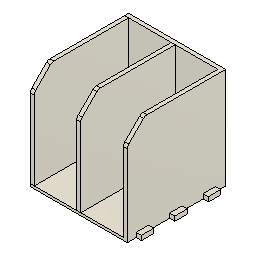
Centerpiece Divider Rack (Autodesk Fusion 360 design; units mm, degrees)
Autodesk Fusion 360 part; units mm, degrees
sketch "Base" plane through (0, 0, 0) normal (0, 1, 0) x (1, 0, 0) in component "DDD Wall Control Center Piece Parametric Template"
  line L0 (36.995, -37.5) -> (-36.995, -37.5)
  line L1 (-36.995, -37.5) -> (-36.995, 37.5)
  line L2 (-36.995, 37.5) -> (36.995, 37.5)
  line L3 (36.995, 37.5) -> (36.995, -37.5)
  line L4 (36.995, -37.5) -> (-36.995, 37.5) construction
  line L5 (-36.995, -37.5) -> (36.995, 37.5) construction
  dimension "d1" = 73.99
  dimension "d2" = 75
  constraint horizontal L0
  constraint perpendicular L0 L1
  constraint parallel L0 L2
  constraint parallel L1 L3
  constraint coincident L4 origin
  constraint coincident L5 origin
  constraint vertical L1
  measures "d1" distance of L1.end L2.end
  measures "d2" distance of L0.end L1.end
extrude "Extrude1" add sketch "Base" along normal blind 2 makes body 1 in component "DDD Wall Control Center Piece Parametric Template"
sketch "Mouting Tab" plane through (0, 0, 0) normal (1, 0, 0) x (0, 0, 1) in component "DDD Wall Control Center Piece Parametric Template"
  line L0 (-20.25, -3.5) -> (-29.75, -3.5)
  line L1 (-29.75, -3.5) -> (-29.75, 0)
  line L2 (-29.75, 0) -> (-20.25, 0)
  line L3 (-20.25, 0) -> (-20.25, -3.5)
  line L4 (-20.25, -3.5) -> (-29.75, 0) construction
  line L5 (-29.75, -3.5) -> (-20.25, 0) construction
  line L6 (1.75, 0) -> (22.5, 0)
  point P0 (-25, -1.75)
  dimension "d34" = 9.5
  dimension "d35" = 3.5
  dimension "d147" = 20.25
  constraint horizontal L0
  constraint perpendicular L0 L1
  constraint parallel L0 L2
  constraint parallel L1 L3
  constraint coincident L4 P0
  constraint coincident L5 P0
  constraint collinear L2 L6
  measures "d34" distance of L1.end L2.end
  measures "d35" distance of L0.end L1.end
  measures "d147" horizontal distance of L2.end origin
extrude "Extrude3" add sketch "Mouting Tab" along normal blind 4 from surface at 36.995 bodies 1 in component "DDD Wall Control Center Piece Parametric Template"
extrude "Extrude6" add sketch "Mouting Tab" against normal blind 4 from surface at -36.995 bodies 1 in component "DDD Wall Control Center Piece Parametric Template"
pattern_linear "R-Pattern2" count 1 spacing 177.59 along (0, -1, 0) count 3 spacing 25.5 along (0, 0, 1) of "Extrude3", "Extrude6" in component "DDD Wall Control Center Piece Parametric Template"
sketch "Side and Back Walls" plane through (0, 2, 0) normal (0, 1, 0) x (-1, 0, 0) in component "DDD Wall Control Center Piece Parametric Template"
  line L0 (-36.995, -37.5) -> (36.995, -37.5)
  line L1 (36.995, -37.5) -> (36.995, 37.5)
  line L2 (36.995, 37.5) -> (-36.995, 37.5)
  line L3 (-36.995, 37.5) -> (-36.995, 30.75)
  line L4 (36.995, -37.5) -> (-36.995, -37.5)
  line L5 (-36.995, -37.5) -> (-36.995, -34.5)
  line L6 (-36.995, -34.5) -> (36.995, -34.5)
  line L7 (36.995, -34.5) -> (36.995, -37.5)
  line L8 (-36.995, 37.5) -> (-33.995, 37.5)
  line L9 (-33.995, 37.5) -> (-33.995, -34.5)
  line L10 (-33.995, -34.5) -> (-36.995, -34.5)
  line L11 (-36.995, -34.5) -> (-36.995, 37.5)
  line L12 (36.995, 37.5) -> (33.995, 37.5)
  line L13 (33.995, 37.5) -> (33.995, -34.5)
  line L14 (33.995, -34.5) -> (36.995, -34.5)
  line L15 (36.995, -34.5) -> (36.995, 37.5)
  line L16 (36.995, -29.75) -> (36.995, -20.25)
  line L17 (36.995, -20.25) -> (36.995, -4.25)
  line L18 (36.995, -4.25) -> (36.995, 5.25)
  line L19 (36.995, 5.25) -> (36.995, 21.25)
  line L20 (36.995, 21.25) -> (36.995, 30.75)
  line L21 (36.995, 30.75) -> (36.995, 37.5)
  line L22 (-36.995, 30.75) -> (-36.995, 21.25)
  line L23 (-36.995, 21.25) -> (-36.995, 5.25)
  line L24 (-36.995, 5.25) -> (-36.995, -4.25)
  line L25 (-36.995, -4.25) -> (-36.995, -20.25)
  line L26 (-36.995, -20.25) -> (-36.995, -29.75)
  line L27 (-36.995, -29.75) -> (-36.995, -37.5)
  dimension "d10" = 3
  dimension "d11" = 3
  dimension "d12" = 3
  constraint horizontal L4
  constraint vertical L5
  constraint horizontal L6
  constraint vertical L7
  constraint coincident L3 L5.end
  constraint coincident L0.end L1.start
  constraint horizontal L8
  constraint vertical L9
  constraint horizontal L10
  constraint vertical L11
  constraint coincident L6 L9.end
  constraint coincident L2.end L3.start
  constraint horizontal L12
  constraint vertical L13
  constraint horizontal L14
  constraint vertical L15
  constraint coincident L6 L13.end
  constraint coincident L1.end L2.start
  measures "d10" distance of L0.start L5.end
  measures "d11" distance of L2.end L8.end
  measures "d12" distance of L1.end L12.end
extrude "Extrude7" add sketch "Side and Back Walls" along normal blind 75 contours L0 L1 L4 L5 L6 L7 L10 L14 L27 | L2 L3 L6 L8 L9 L10 L11 L22 L23 L24 L25 L26 L27 | L1 L2 L6 L12 L13 L14 L15 L16 L17 L18 L19 L20 L21 bodies 1 in component "DDD Wall Control Center Piece Parametric Template"
extrude "Extrude11" add sketch "Side and Back Walls" along normal blind 75 separate body contours L1 L2 L6 L12 L13 L14 L15 L16 L17 L18 L19 L20 L21 makes body 2 in component "DDD Wall Control Center Piece Parametric Template"
sketch "Divider Wall" plane through (-33.995, 0, 0) normal (1, 0, 0) x (0, 0, -1) in component "DDD Wall Control Center Piece Parametric Template"
  line L0 (-37.5, 2) -> (34.5, 2)
  line L1 (34.5, 2) -> (34.5, 77)
  line L2 (34.5, 77) -> (-37.5, 77)
  line L3 (-37.5, 77) -> (-37.5, 2)
  line L4 (-22.5, 77) -> (-18.75, 77)
  line L5 (-18.75, 77) -> (-18.75, 58.25)
  line L6 (-18.75, 58.25) -> (-37.5, 58.25)
  line L7 (-37.5, 58.25) -> (-37.5, 62)
  line L8 (-25.1517, 75.9017) -> (-36.4017, 64.6517)
  arc A0 (-22.5, 77) -> (-25.1517, 75.9017) centre (-22.5, 73.25) ccw
  arc A1 (-36.4017, 64.6517) -> (-37.5, 62) centre (-33.75, 62) ccw
  dimension "d59" = 18.75
  dimension "d60" = 18.75
  dimension "d62" = 18.75
  dimension "d63" = 18.75
  dimension "d70" = 3.75
  dimension "d71" = 3.75
  dimension "d72" = 3.75
  dimension "d73" = 3.75
  constraint horizontal L4
  constraint vertical L5
  constraint horizontal L6
  constraint vertical L7
  constraint tangent L4 A0
  constraint tangent L8 A0
  constraint tangent L7 A1
  constraint tangent L8 A1
  measures "d59" distance of L4.end L5.end
  measures "d60" distance of L5.end L6.end
  measures "d62" distance of L3 L5
  measures "d63" distance of L2 L6
  measures "d70" radius of A0
  measures "d71" radius of A1
  measures "d72" distance of L4.end L4.start
  measures "d73" distance of L6.end L7.end
extrude "Extrude12" cut sketch "Divider Wall" along normal up to surface (-3 mm away) and the other way up to surface (-70.99 mm away) contours L2 L3 L8 A0 A1 bodies 1 2 in component "DDD Wall Control Center Piece Parametric Template"
pattern_linear "R-Pattern3" count 1 spacing 0 along (0, -1, 0) count 2 spacing 35.495 along (1, 0, 0) of bodies 2 makes body 3 in component "DDD Wall Control Center Piece Parametric Template"
component "Divider Rack" placed x (1, 0, 0) y (0, 1, 0) z (0, 0, 1) at (0, 0, 0)
component "DDD Wall Control Center Piece Parametric Template" placed x (1, 0, 0) y (0, 1, 0) z (0, 0, 1) at (0, 0, 0) in component "Divider Rack"
equation "d1 = MMCenterPieceWidth"
equation "d2 = CenterPieceDepth"
equation "d3 = CenterPieceThickness"
equation "CenterPieceWidthUnits = 3" comment "Number of width spaces on the wall control pegboard.  Minimum 1,  maximum 14 for vertical wall control panels,  and 31 for horizonal panels.  Realistically your printer dimensions will determin how big you can make this."
equation "MMCenterPieceWidth = ( CenterPieceWidthUnits * 25.4 mm ) - 2.21 mm" comment "Don't change this.  Change CenterPieceWidthUnits instead.  Final width dimension subtracts 2.21mm from the standard 1\" space between wall control slots to account for the tabs for mouting into the slots"
equation "CenterPieceDepth = 75 mm" comment "Depth measurement from the wall control board extending out into space.  Minimum 17mm to fit at least one mounting tab.  Maximum  ¯\\_(ツ)_/¯"
equation "CenterPieceThickness = 2 mm" comment "Lower measurements make for good shelf-like objects,  taller measurement make for better custom tool holders"
equation "d147 = CenterPieceDepth / 2 - 17.25 mm"
equation "CountMountingTabs = 3" comment "Specify the number of mounting tabs to attach a sidepiece"
equation "d150 = CountMountingTabs"
equation "DividerWallThickness = 3 mm" comment "Specify the thickness of the divider walls (including the outter side and back walls)"
equation "d10 = DividerWallThickness"
equation "d11 = DividerWallThickness"
equation "d12 = DividerWallThickness"
equation "DividerWallHeigth = 75 mm" comment "Specify how tall the divider walls should be (including the outter side and back walls)"
equation "d14 = DividerWallHeigth"
equation "DividerWallBevel = DividerWallHeigth - ( DividerWallHeigth * 0.75 )" comment "Don't change this.  Calculates the percentage of the divider wall height to use as the bevel radius measurment"
equation "d51 = DividerWallHeigth"
equation "d54 = DividerWallCount"
equation "d56 = -DividerWallSpacing"
equation "DividerWallCount = 2" comment "Specify the number of divider walls.  Minimum 2 (one is always combined inside a side wall).  Maximum  ¯\\_(ツ)_/¯"
equation "DividerWallSpacing = ( MMCenterPieceWidth - DividerWallThickness ) / DividerWallCount" comment "Don't change this.  Calculates the spacing between the divider walls based on how many are specified in DividerWallCount"
equation "d59 = DividerWallBevel"
equation "d60 = DividerWallBevel"
equation "d62 = DividerWallBevel"
equation "d63 = DividerWallBevel"
equation "MeasurementBetweenWalls = DividerWallSpacing - DividerWallThickness" comment "Unused.  Provided here so you can see if your tools will fit between the walls."
equation "HowToUse = 0" comment "Insert this into a new design, and then break the link to the original to preserve the template.  Then modify as needed for centerpiece tool holders."
equation "d70 = DividerWallBevel / 5"
equation "d71 = DividerWallBevel / 5"
equation "d72 = DividerWallBevel / 5"
equation "d73 = DividerWallBevel / 5"
named bodies: "Center Piece Parametric Template", "Divider Wall", "Divider Wall (1)"
